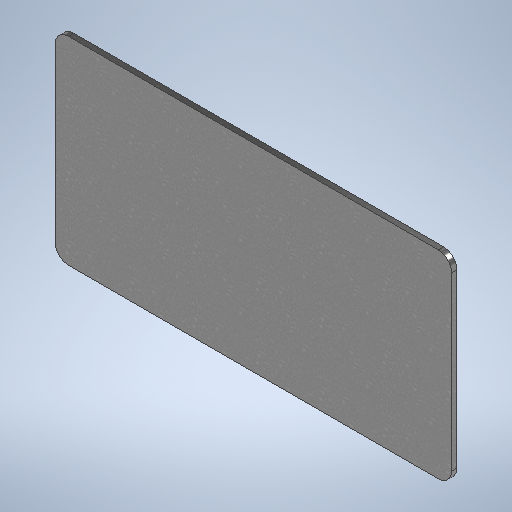
# Autodesk Inventor part: Sessao5_0001_001
Saved by Autodesk Inventor 2025.2 (Build 292293000, 293)
## iProperties
Created: 2025-03-28
Part Number: Sessao5_0001_001
Material: Aço, fundido
Document SubType Name: Sheet Metal
Designer: lucas
Density: 7.85 g/cm^3
Sheet Metal Rule: Padrão_mm
Appearance: Aço galvanizado
Author: lucas
Autodesk Inventor part; units mm, degrees
ref_plane "YZ Plane" through (0, 0, 0) normal (1, 0, 0) x (0, 1, 0)
ref_plane "XZ Plane" through (0, 0, 0) normal (0, 1, 0) x (-1, 0, 0)
ref_plane "XY Plane" through (0, 0, 0) normal (0, 0, 1) x (1, 0, 0)
sketch "Esboço1" plane through (0, 0, 0) normal (0, 0, 1) x (1, 0, 0)
  line L0 (-750, -375) -> (750, -375)
  line L1 (750, -375) -> (750, 375)
  line L2 (750, 375) -> (-750, 375)
  line L3 (-750, 375) -> (-750, -375)
  line L4 (-750, -375) -> (750, 375) construction
  line L5 (750, -375) -> (-750, 375) construction
  point P0 (0, 0)
  dimension "d0" = 1500
  dimension "d1" = 750
  measures "d0" distance of L2.end L1.end
  measures "d1" distance of L1.end L0.end
extrude "Placa1" add sketch "Esboço1" along normal mid plane 20
fillet "Arredondamento1" radius 50 1 edges at (-750, 375, 0)
fillet "Arredondamento2" radius 50 2 edges at (750, 375, 0) (750, -375, 0)
fillet "Arredondamento3" radius 50 1 edges at (-750, -375, 0)
equation "\"d2\" = Espessura"
equation "\"Espessura\" = 20"
